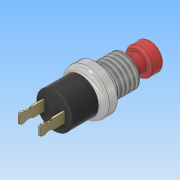
# Autodesk Inventor part: Push Button
Saved by Autodesk Inventor 2019 (Build 230136000, 136)
## iProperties
Created: 2021-05-06
Part Number: Push Button
Material: Generic
Document SubType Name: Modeling
Designer: David
Density: 1 g/cm^3
Appearance: Default
Author: David
Autodesk Inventor part; units mm, degrees
ref_plane "YZ Plane" through (0, 0, 0) normal (1, 0, 0) x (0, 1, 0)
ref_plane "XZ Plane" through (0, 0, 0) normal (0, 1, 0) x (-1, 0, 0)
ref_plane "XY Plane" through (0, 0, 0) normal (0, 0, 1) x (1, 0, 0)
sketch "Sketch1" plane through (0, 0, 0) normal (0, 0, 1) x (1, 0, 0)
  circle A0 centre (0, 0) radius 4
  dimension "d0" = 8
  constraints: 1 centre point, 1 coincident
  measures "d0" diameter of A0
extrude "Extrusion1" add sketch "Sketch1" along normal blind 6
sketch "Sketch2" plane through (0, 0, 6) normal (0, 0, 1) x (1, 0, 0)
  line L0 (2.1, 1.125) -> (2.5, 1.125)
  line L1 (2.5, 1.125) -> (2.5, -1.125)
  line L2 (2.5, -1.125) -> (2.1, -1.125)
  line L3 (2.1, -1.125) -> (2.1, 1.125)
  line L4 (-2.5, 1.125) -> (-2.1, 1.125)
  line L5 (-2.1, 1.125) -> (-2.1, -1.125)
  line L6 (-2.1, -1.125) -> (-2.5, -1.125)
  line L7 (-2.5, -1.125) -> (-2.5, 1.125)
  point P0 (0, 0)
  point P1 (2.1, 0)
  point P2 (-2.5, 0)
  dimension "d3" = 2.25
  dimension "d6" = 2.25
  dimension "d9" = 0.4
  dimension "d10" = 0.4
  dimension "d11" = 2.5
  dimension "d12" = 2.5
  constraints: 16 end point, 4 parallel, 2 horizontal, 2 midpoint, 2 perpendicular, 1 horizontal alignment
  measures "d3" distance of L0.end L1.end
  measures "d6" distance of L4.end L5.end
  measures "d9" distance of L5.end L6.end
  measures "d10" distance of L1.end L2.end
  measures "d11" distance from line of L1 point (0, 0)
  measures "d12" distance from line of point (0, 0) L7
extrude "Extrusion2" add sketch "Sketch2" along normal blind 5.5
sketch "Sketch3" plane through (2.5, -1.125, 6) normal (1, 0, 0) x (0, 0, -1)
  line L0 (0, 2.25) -> (-5.5, 2.25) projected
  line L1 (0, 2.25) -> (-2.5, 2.25)
  arc A0 (-4.5, 2.25) -> (-2.5, 2.25) centre (-3.5, 3.549) ccw
  line L2 (-5.5, 0) -> (-5.5, 2.25) projected
  line L3 (-5.5, 1.125) -> (-5.2177, 1.125)
  arc A1 (-5.1597, 2.25) -> (-5.5, 1.9097) centre (-5.1597, 1.9097) ccw
  line L4 (-5.5, 1.9097) -> (-5.1597, 2.25) construction
  line L5 (-5.5, 1.9097) -> (-5.0187, 1.9097) construction
  line L6 (-5.5, 1.125) -> (-5.5, 1.9097)
  line L7 (-5.1597, 2.25) -> (-4.5, 2.25)
  arc A2 (-2.5, 0) -> (-4.5, 0) centre (-3.5, -1.299) ccw
  arc A3 (-5.5, 0.3403) -> (-5.1597, 0) centre (-5.1597, 0.3403) ccw
  line L8 (0, 0) -> (-5.5, 0) projected
  line L9 (-5.5, 0.3403) -> (-5.5, 0)
  line L10 (-5.5, 0) -> (-5.1597, 0)
  line L11 (-4.5, 0) -> (-2.5, 0)
  point P0 (6, 1.125)
  dimension "d15" = 2.5
  dimension "d16" = 2
  dimension "d17" = 45
  constraints: 18 end point, 8 point on circle, 6 symmetric about line, 4 centre point, 4 point on line, 3 collinear, 2 horizontal, 2 perpendicular, 2 tangent, 1 equal length, 1 midpoint, 2 other
  measures "d15" distance of L0.start L1.end
  measures "d16" distance of L1.end L7.end
  measures "d17" angle of L5 L4
extrude "Extrusion3" cut sketch "Sketch3" against normal up to surface (5 mm away)
sketch "Sketch4" plane through (0, 0, 0) normal (0, 1, 0) x (-1, 0, 0)
  line L0 (0, 0) -> (0, -3.2)
  line L1 (0, -3.2) -> (5, -3.2)
  line L2 (5, -3.2) -> (5, -1.4)
  line L3 (-4, 0) -> (4, 0) projected
  arc A0 (5, -1.4404) -> (4, 0) centre (3.4626, -1.4404) ccw
  line L4 (4, 0) -> (0, 0)
  dimension "d20" = 3.2
  dimension "d21" = 5
  dimension "d22" = 1.8
  constraints: 8 end point, 2 point on circle, 2 vertical, 1 centre point, 1 collinear, 1 horizontal, 1 point on line, 1 tangent
  measures "d20" distance of L0.start L0.end
  measures "d21" distance of L0.end L1.end
  measures "d22" distance of L1.end L2.end
revolve "Revolution1" add sketch "Sketch4" angle 360 about axis through (0, 0, 0) along (0, 0, -1)
sketch "Sketch5" plane through (0, 0, -3.2) normal (0, 0, -1) x (-1, 0, 0)
  circle A0 centre (0, 0) radius 3.5
  dimension "d24" = 7
  constraints: 1 centre point, 1 coincident
  measures "d24" diameter of A0
extrude "Extrusion4" add sketch "Sketch5" along normal blind 1.5
sketch "Sketch7" plane through (0, 0, -4.7) normal (0, 0, -1) x (-1, 0, 0)
  circle A0 centre (0, 0) radius 3.525
  dimension "d29" = 7.05
  constraints: 1 centre point, 1 coincident
  measures "d29" diameter of A0
extrude "Extrusion6" add sketch "Sketch7" along normal blind 5
thread "Thread1" size "M6x1" class "6g" standard "ANSI Metric M Profile" length 10
sketch "Sketch8" plane through (0, 0, -9.7) normal (0, 0, -1) x (-1, 0, 0)
  circle A0 centre (0, 0) radius 2
  dimension "d34" = 4
  constraints: 1 centre point, 1 coincident
  measures "d34" diameter of A0
extrude "Extrusion7" add sketch "Sketch8" along normal blind 3
sketch "Sketch9" plane through (0, 0, -12.7) normal (0, 0, -1) x (-1, 0, 0)
  circle A0 centre (0, 0) radius 3
  dimension "d37" = 6
  constraints: 1 centre point, 1 coincident
  measures "d37" diameter of A0
extrude "Extrusion8" add sketch "Sketch9" along normal blind 3
fillet "Fillet1" radius 0.5 2 edges at (3, 0, -12.7) (3, 0, -15.7)
fillet "Fillet2" radius 0.2 1 edges at (-4, 0, 6)
equation "\"d9\" = d10"
equation "\"d12\" = d11"
body "Solid1"
